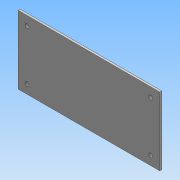
# Autodesk Inventor part: Heater_pcb
Saved by Autodesk Inventor 2016 (Build 200138000, 138)
## iProperties
Created: 2016-04-03
Part Number: Heater_pcb
Material: Generic
Document SubType Name: Modeling
Designer: admin
Density: 1 g/cm^3
Appearance: Default
Author: admin
Autodesk Inventor part; units mm, degrees
ref_plane "YZ Plane" through (0, 0, 0) normal (1, 0, 0) x (0, 1, 0)
ref_plane "XZ Plane" through (0, 0, 0) normal (0, 1, 0) x (-1, 0, 0)
ref_plane "XY Plane" through (0, 0, 0) normal (0, 0, 1) x (1, 0, 0)
sketch "Sketch1" plane through (0, 0, 0) normal (0, 1, 0) x (-1, 0, 0)
  line L0 (55, -26.5) -> (-55, -26.5)
  line L1 (-55, -26.5) -> (-55, 26.5)
  line L2 (-55, 26.5) -> (55, 26.5)
  line L3 (55, 26.5) -> (55, -26.5)
  point P0 (0, 0)
  point P1 (0, -26.5)
  point P2 (55, 0)
  dimension "d0" = 53
  dimension "d1" = 110
  constraints: 8 end point, 2 midpoint, 2 parallel, 1 horizontal, 1 horizontal alignment, 1 perpendicular, 1 vertical alignment
  measures "d0" distance of L0.end L1.end
  measures "d1" distance of L0.start L0.end
extrude "Extrusion1" add sketch "Sketch1" along normal blind 1.6
sketch "Sketch2" plane through (0, 1.6, 0) normal (0, 1, 0) x (1, 0, 0)
  line L0 (55, 26.5) -> (-55, 26.5) projected
  line L1 (-55, 26.5) -> (-55, -26.5) projected
  line L2 (-55, -26.5) -> (55, -26.5) projected
  line L3 (55, -26.5) -> (55, 26.5) projected
  point P0 (0, 0)
  point P1 (-48, -19.5)
  point P2 (-48, 19.5)
  point P3 (48, -19.5)
  point P4 (48, 19.5)
  dimension "d4" = 7
  dimension "d5" = 7
  dimension "d6" = 7
  dimension "d7" = 7
  constraints: 2 horizontal alignment, 2 vertical alignment
  measures "d4" distance from line of L3 point (48, 19.5)
  measures "d5" distance from line of L0 point (48, 19.5)
  measures "d6" distance from line of L1 point (-48, -19.5)
  measures "d7" distance from line of L2 point (-48, -19.5)
hole "Hole1" at (-48, 1.6, 19.5) at (-48, 1.6, -19.5) at (48, 1.6, 19.5) at (48, 1.6, -19.5) direction (0, -1, 0) diameter 3 end through all
equation "\"d5\" = d4"
equation "\"d6\" = d4"
equation "\"d7\" = d4"
body "Solid1"
